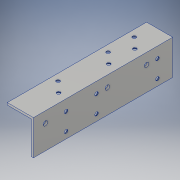
# Autodesk Inventor part: CLB_086_ClimberMountLowerAngle
Saved by Autodesk Inventor 2018.3 (Build 223284000, 284)
## iProperties
Created: 2020-02-22
Part Number: CLB_086_ClimberMountLowerAngle
Material: Aluminum 6061
Document SubType Name: Modeling
Designer: 22perngrac
Density: 2.7 g/cm^3
Appearance: Aluminum - Flat
Mass: 146.982 g
Surface Area: 368.225 cm^2
Volume: 54.4379 cm^3
Author: 22perngrac
Autodesk Inventor part; units mm, degrees
ref_plane "YZ Plane" through (0, 0, 0) normal (1, 0, 0) x (0, 1, 0)
ref_plane "XZ Plane" through (0, 0, 0) normal (0, 1, 0) x (-1, 0, 0)
ref_plane "XY Plane" through (0, 0, 0) normal (0, 0, 1) x (1, 0, 0)
sketch "Sketch1" plane through (0, 0, 0) normal (0, 0, 1) x (1, 0, 0)
  line L0 (0, 0) -> (38.1, 0)
  line L1 (38.1, 0) -> (38.1, -50.8)
  line L2 (38.1, -50.8) -> (34.925, -50.8)
  line L3 (34.925, -50.8) -> (34.925, -3.175)
  line L4 (34.925, -3.175) -> (0, -3.175)
  line L5 (0, -3.175) -> (0, 0)
  dimension "d0" = 50.8
  dimension "d1" = 38.1
  dimension "d2" = 3.175
  dimension "d3" = 3.175
  constraints: 12 end point, 5 perpendicular, 1 horizontal
  measures "d0" distance of L0.end L1.end
  measures "d1" distance of L0.start L0.end
  measures "d2" distance between parallel lines of L4 L0
  measures "d3" distance between parallel lines of L1 L3
extrude "Extrusion1" add sketch "Sketch1" along normal blind 203.2
sketch "Sketch2" plane through (0, -3.175, 0) normal (0, 1, 0) x (1, 0, 0)
  line L0 (38.1, -203.2) -> (0, -203.2) projected
  line L1 (38.1, 0) -> (38.1, -203.2) projected
  line L2 (0, 0) -> (0, -203.2) projected
  line L3 (0, 0) -> (38.1, 0) projected
  point P0 (25.2222, -153.4922)
  point P1 (9.9314, -139.0904)
  point P2 (25.2222, -80.4672)
  point P3 (9.9314, -66.0654)
  point P4 (25.2222, -42.3672)
  point P5 (9.9314, -27.9654)
  dimension "d6" = 49.7078
  dimension "d8" = 9.9314
  dimension "d9" = 64.1096
  dimension "d10" = 25.2222
  dimension "d11" = 80.4672
  dimension "d12" = 25.2222
  dimension "d13" = 66.0654
  dimension "d14" = 9.9314
  dimension "d15" = 42.3672
  dimension "d16" = 25.2222
  dimension "d17" = 27.9654
  dimension "d18" = 9.9314
  measures "d6" distance from line of point (25.222, -153.492) L0
  measures "d8" distance from line of L2 point (9.931, -139.09)
  measures "d9" distance from line of L0 point (9.931, -139.09)
  measures "d10" distance from line of L2 point (25.222, -153.492)
  measures "d11" distance from line of L3 point (25.222, -80.467)
  measures "d12" distance from line of L2 point (25.222, -80.467)
  measures "d13" distance from line of L3 point (9.931, -66.065)
  measures "d14" distance from line of L2 point (9.931, -66.065)
  measures "d15" distance from line of L3 point (25.222, -42.367)
  measures "d16" distance from line of L2 point (25.222, -42.367)
  measures "d17" distance from line of L3 point (9.931, -27.965)
  measures "d18" distance from line of L2 point (9.931, -27.965)
hole "Hole1" at (25.2222, -3.175, 153.4922) at (9.9314, -3.175, 139.0904) at (25.2222, -3.175, 80.4672) at (9.9314, -3.175, 66.0654) at (25.2222, -3.175, 42.3672) at (9.9314, -3.175, 27.9654) direction (0, 1, 0) diameter 5.1054 end through all countersink diameter 9.525 countersink angle 82
sketch "Sketch4" plane through (34.925, -50.8, 0) normal (1, 0, 0) x (0, 0, -1)
  line L0 (0, 50.8) -> (0, 0) projected
  line L1 (0, 50.8) -> (-203.2, 50.8) projected
  line L2 (-203.2, 0) -> (-203.2, 50.8) projected
  point P0 (-22.225, 34.925)
  point P1 (-22.225, 9.525)
  point P2 (-155.575, 34.925)
  point P3 (-155.575, 9.525)
  point P4 (-111.125, 34.925)
  point P5 (-111.125, 9.525)
  dimension "d29" = 25.4
  dimension "d30" = 22.225
  dimension "d31" = 22.225
  dimension "d32" = 15.875
  dimension "d33" = 47.625
  dimension "d34" = 47.625
  dimension "d35" = 25.4
  dimension "d36" = 15.875
  dimension "d41" = 92.075
  dimension "d42" = 92.075
  dimension "d43" = 25.4
  dimension "d44" = 15.875
  measures "d29" distance of point (-22.225, 9.525) point (-22.225, 34.925)
  measures "d30" distance from line of L0 point (-22.225, 34.925)
  measures "d31" distance from line of L0 point (-22.225, 9.525)
  measures "d32" distance from line of point (-22.225, 34.925) L1
  measures "d33" distance from line of L2 point (-155.575, 34.925)
  measures "d34" distance from line of L2 point (-155.575, 9.525)
  measures "d35" distance of point (-155.575, 9.525) point (-155.575, 34.925)
  measures "d36" distance from line of point (-155.575, 34.925) L1
  measures "d41" distance from line of L2 point (-111.125, 34.925)
  measures "d42" distance from line of L2 point (-111.125, 9.525)
  measures "d43" distance of point (-111.125, 9.525) point (-111.125, 34.925)
  measures "d44" distance from line of point (-111.125, 34.925) L1
hole "Hole2" at (34.925, -15.875, 22.225) at (34.925, -41.275, 22.225) at (34.925, -15.875, 155.575) at (34.925, -41.275, 155.575) at (34.925, -15.875, 111.125) at (34.925, -41.275, 111.125) direction (1, 0, 0) diameter 5.1054 end through all countersink diameter 9.779 countersink angle 82 clearance for "Flat Head Machine Screw (82)" size "#10" standard "Ansi Unified Screw Threads"
sketch "Sketch5" plane through (34.925, -50.8, 0) normal (-1, 0, 0) x (0, 0, 1)
  line L0 (0, 47.625) -> (203.2, 47.625) projected
  line L1 (0, 0) -> (0, 47.625) projected
  point P0 (0, 50.8)
  point P1 (38.1, 34.925)
  point P2 (95.25, 34.925)
  point P3 (185.7899, 34.925)
  dimension "d52" = 12.7
  dimension "d53" = 38.1
  dimension "d54" = 95.25
  dimension "d55" = 185.7899
  constraints: 2 horizontal alignment
  measures "d52" distance from line of point (38.1, 34.925) L0
  measures "d53" distance from line of point (38.1, 34.925) L1
  measures "d54" distance from line of point (95.25, 34.925) L1
  measures "d55" distance from line of point (185.79, 34.925) L1
hole "Hole3" at (34.925, -15.875, 38.1) at (34.925, -15.875, 95.25) at (34.925, -15.875, 185.7899) direction (1, 0, 0) diameter 6.35 end through all
equation "\"d3\" = d2"
equation "\"d31\" = d30"
equation "\"d34\" = d33"
equation "\"d42\" = d41"
body "Solid1"
